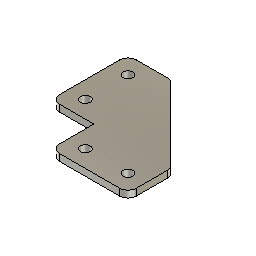
Project Cart v3 v1 (Autodesk Fusion 360 archive; units mm, degrees)
design "Corner Bracket Shelf Support"
Autodesk Fusion 360 part; units mm, degrees
note: some values were not read from the file. Set by a fixed rule: the direction of a hole.
sketch "Bracket Shape" plane through (0, 0, 0) normal (0, 0, 1) x (1, 0, 0) in component "Bracket"
  line L0 (0, 0) -> (70, 0)
  line L1 (70, 0) -> (70, 70)
  line L2 (70, 70) -> (0, 70)
  line L3 (0, 70) -> (0, 0)
  line L4 (0, 0) -> (25, 0)
  line L5 (25, 0) -> (25, 25)
  line L6 (25, 25) -> (0, 25)
  line L7 (0, 25) -> (0, 0)
  line L8 (25, 25) -> (25, 70)
  line L9 (25, 25) -> (70, 25)
  line L10 (25, 70) -> (70, 25)
  line L11 (0, 70) -> (10, 70)
  line L12 (10, 70) -> (10, 25) construction
  line L13 (70, 0) -> (70, 10) construction
  line L14 (70, 10) -> (25, 10) construction
  line L15 (70, 0) -> (60, 0) construction
  line L16 (25, 0) -> (35, 0) construction
  line L17 (35, 0) -> (35, 10) construction
  line L18 (60, 0) -> (60, 10) construction
  line L19 (0, 25) -> (0, 35) construction
  line L20 (0, 70) -> (0, 60) construction
  line L21 (0, 70) -> (0, 60) construction
  line L22 (0, 35) -> (10, 35) construction
  line L23 (0, 60) -> (10, 60) construction
  line L24 (25, 10) -> (0, 10) construction
  line L25 (10, 25) -> (10, 0) construction
  dimension "d1" = 70
  dimension "d2" = 70
  dimension "d3" = 25
  dimension "d4" = 25
  dimension "d7" = 10
  dimension "d8" = 10
  dimension "d9" = 10
  dimension "d10" = 10
  dimension "d11" = 10
  dimension "d12" = 10
  constraint horizontal L0
  constraint vertical L1
  constraint horizontal L2
  constraint vertical L3
  constraint coincident L0.start L3.end
  constraint horizontal L4
  constraint vertical L5
  constraint horizontal L6
  constraint vertical L7
  constraint coincident L2 L8.end
  constraint perpendicular L2 L8
  constraint coincident L1 L9.end
  constraint perpendicular L1 L9
  constraint perpendicular L3 L11
  constraint coincident L6 L12.end
  constraint perpendicular L6 L12
  constraint perpendicular L0 L13
  constraint coincident L5 L14.end
  constraint perpendicular L5 L14
  constraint perpendicular L1 L15
  constraint perpendicular L5 L16
  constraint coincident L14 L17.end
  constraint perpendicular L14 L17
  constraint coincident L14 L18.end
  constraint perpendicular L14 L18
  constraint perpendicular L6 L19
  constraint coincident L3 L20.end
  constraint perpendicular L11 L21
  constraint coincident L12 L22.end
  constraint perpendicular L12 L22
  constraint coincident L12 L23.end
  constraint perpendicular L12 L23
  constraint coincident L7 L24.end
  constraint coincident L4 L25.end
  measures "d1" distance of L1.end L2.end
  measures "d2" distance of L0.end L1.end
  measures "d3" distance of L4.end L5.end
  measures "d4" distance of L5.end L6.end
  measures "d7" distance of L2.end L11.end
  measures "d8" distance of L0.end L13.end
  measures "d9" distance of L0.end L15.end
  measures "d10" distance of L4.end L16.end
  measures "d11" distance of L6.end L19.end
  measures "d12" distance of L2.end L20.end
extrude "Extrude1" add sketch "Bracket Shape" along normal blind 4 contours L0 L1 L5 L9 | L2 L3 L6 L8 L11 | L8 L9 L10 in component "Bracket"
hole "Hole1" at (10, 60, 0) direction (0, 0, 1) diameter 5.8 end through all in component "Bracket"
hole "Hole2" at (10, 35, 0) direction (0, 0, 1) diameter 5.8 end through all in component "Bracket"
hole "Hole3" at (35, 10, 0) direction (0, 0, 1) diameter 5.8 end through all in component "Bracket"
hole "Hole4" at (60, 10, 0) direction (0, 0, 1) diameter 5.8 end through all in component "Bracket"
fillet "Fillet1" radius 5 6 edges at (70, 0, 2) (25, 0, 2) (0, 25, 2) (0, 70, 2) (25, 70, 2) (70, 25, 2) in component "Bracket"
component "Bracket" placed x (1, 0, 0) y (0, 1, 0) z (0, 0, 1) at (0, 0, 0)
